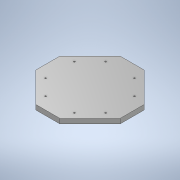
# Autodesk Inventor part: Base
Saved by Autodesk Inventor 2021 (Build 250183000, 183)
## iProperties
Created: 2021-03-02
Part Number: Base
Material: Plástico ABS
Document SubType Name: Modeling
Designer: Marc
Density: 1.06 g/cm^3
Appearance: Suave - Blanco
Author: Marc
Autodesk Inventor part; units mm, degrees
ref_plane "YZ Plane" through (0, 0, 0) normal (1, 0, 0) x (0, 1, 0)
ref_plane "XZ Plane" through (0, 0, 0) normal (0, 1, 0) x (-1, 0, 0)
ref_plane "XY Plane" through (0, 0, 0) normal (0, 0, 1) x (1, 0, 0)
sketch "Boceto1" plane through (0, 0, 0) normal (0, 1, 0) x (-1, 0, 0)
  line L0 (-87.5, 87.5) -> (87.5, -87.5) construction
  line L1 (87.5, 87.5) -> (-87.5, -87.5) construction
  line L2 (-87.5, -25) -> (-87.5, 25)
  line L3 (-87.5, 25) -> (-25, 87.5)
  line L4 (-25, 87.5) -> (25, 87.5)
  line L5 (25, 87.5) -> (87.5, 25)
  line L6 (87.5, -25) -> (25, -87.5)
  line L7 (25, -87.5) -> (-25, -87.5)
  line L8 (-25, -87.5) -> (-87.5, -25)
  line L9 (87.5, -25) -> (87.5, 25)
  circle A0 centre (-62.5, -30) radius 1.5
  circle A1 centre (-62.5, 30) radius 1.5
  circle A2 centre (-30, 62.5) radius 1.5
  circle A3 centre (30, 62.5) radius 1.5
  circle A4 centre (62.5, 30) radius 1.5
  circle A5 centre (62.5, -30) radius 1.5
  circle A6 centre (30, -62.5) radius 1.5
  circle A7 centre (-30, -62.5) radius 1.5
  point P0 (0, 0)
  dimension "d30" = 175
  dimension "d31" = 175
  dimension "d40" = 3
  dimension "d41" = 3
  dimension "d42" = 3
  dimension "d43" = 3
  dimension "d44" = 3
  dimension "d45" = 3
  dimension "d46" = 3
  dimension "d47" = 3
  constraints: 20 end point, 8 centre point, 2 midpoint, 1 vertical
  measures "d30" distance of L0.end L1.end
  measures "d31" distance of L1.start L0.end
  measures "d40" diameter of A0
  measures "d41" diameter of A1
  measures "d42" diameter of A2
  measures "d43" diameter of A3
  measures "d44" diameter of A4
  measures "d45" diameter of A5
  measures "d46" diameter of A6
  measures "d47" diameter of A7
extrude "Extrusión1" add sketch "Boceto1" along normal blind 10
